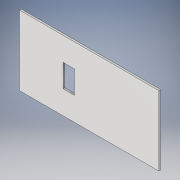
# Autodesk Inventor part: Rt window
Saved by Autodesk Inventor 2017 (Build 210142000, 142)
## iProperties
Created: 2017-06-23
Part Number: Rt window
Material: Generic
Document SubType Name: Modeling
Designer: cas7
Density: 1 g/cm^3
Appearance: Default
Author: cas7
Autodesk Inventor part; units mm, degrees
ref_plane "YZ Plane" through (0, 0, 0) normal (1, 0, 0) x (0, 1, 0)
ref_plane "XZ Plane" through (0, 0, 0) normal (0, 1, 0) x (-1, 0, 0)
ref_plane "XY Plane" through (0, 0, 0) normal (0, 0, 1) x (1, 0, 0)
sketch "Sketch1" plane through (0, 0, 0) normal (0, 0, 1) x (1, 0, 0)
  line L0 (0, 0) -> (1219.2, 0)
  line L1 (1219.2, 0) -> (1219.2, 609.6)
  line L2 (1219.2, 609.6) -> (0, 609.6)
  line L3 (0, 609.6) -> (0, 0)
  line L4 (0, 609.6) -> (0, 0)
  line L5 (382.6, 304.8) -> (382.6, 404.8)
  line L6 (382.6, 404.8) -> (482.6, 404.8)
  line L7 (482.6, 404.8) -> (482.6, 204.8)
  line L8 (482.6, 204.8) -> (382.6, 204.8)
  line L9 (382.6, 204.8) -> (382.6, 304.8)
  dimension "d0" = 1219.2
  dimension "d1" = 609.6
  dimension "d4" = 100
  dimension "d5" = 100
  dimension "d6" = 200
  dimension "d7" = 100
  constraints: 20 end point, 3 equal length, 3 perpendicular, 1 horizontal, 1 point on line
  measures "d0" distance of L2.end L1.end
  measures "d1" distance of L1.end L0.end
  measures "d4" distance of L5.start L5.end
  measures "d5" distance of L5.end L6.end
  measures "d6" distance of L6.end L7.end
  measures "d7" distance of L7.end L8.end
extrude "Extrusion1" add sketch "Sketch1" along normal blind 15.875
body "Solid1"
